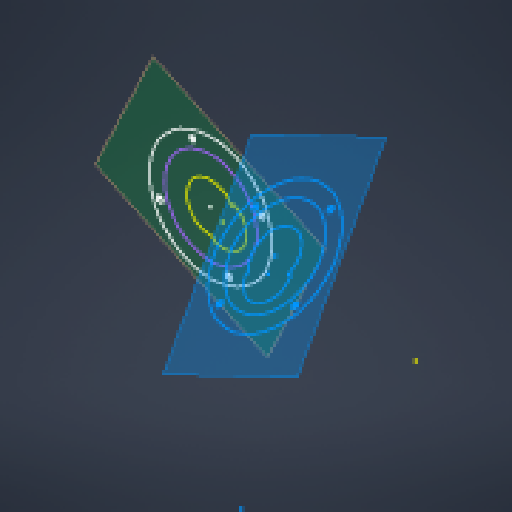
# Autodesk Inventor part: pylon_actuator_holder
Saved by Autodesk Inventor 2023.2 (Build 272271000, 271)
## iProperties
Created: 2023-07-02
Part Number: pylon_actuator_holder
Material: Generic
Document SubType Name: Modeling
Designer: Bober
Density: 1 g/cm^3
Appearance: Default
Author: Bober
Autodesk Inventor part; units mm, degrees
ref_plane "YZ Plane" through (0, 0, 0) normal (1, 0, 0) x (0, 1, 0)
ref_plane "XZ Plane" through (0, 0, 0) normal (0, 1, 0) x (-1, 0, 0)
ref_plane "XY Plane" through (0, 0, 0) normal (0, 0, 1) x (1, 0, 0)
ref_plane "Work Plane1" through (-137.7012, 21.7952, -38) normal (0, 0, -1) x (0.4270356, 0.9042348, 0)
sketch "Sketch1" plane through (-137.7012, 21.7952, -38) normal (0, 0, -1) x (0.4270356, 0.9042348, 0)
  arc A0 (-14.9525, 13.2962) -> (-14.999, 13.2194) centre (0, 4.2038) ccw projected
  arc A1 (14.999, 13.2194) -> (14.9525, 13.2962) centre (0, 4.2038) ccw projected
  circle A2 centre (0, 4.2038) radius 40 projected
  circle A3 centre (-24.7487, 28.9525) radius 2 projected
  circle A4 centre (24.7487, 28.9525) radius 2 projected
  circle A5 centre (24.7487, -20.5449) radius 2 projected
  circle A6 centre (-24.7487, -20.5449) radius 2 projected
  circle A7 centre (0, 4.2038) radius 40
  circle A8 centre (-24.7487, -20.5449) radius 2
  circle A9 centre (-24.7487, 28.9525) radius 2
  circle A10 centre (24.7487, 28.9525) radius 2
  circle A11 centre (24.7487, -20.5449) radius 2
  circle A12 centre (0, 4.2038) radius 30
  point P0 (39.0954, 133.8216)
  dimension "d0" = 3
  constraints: 6 centre point, 6 coincident, 5 concentric
ref_plane "Work Plane2" through (-187.1508, -33.2508, -28) normal (0, 0, 1) x (0.9042348, -0.4270356, 0)
extrude "Extrusion1" add sketch "Sketch1" against normal up to surface (10 mm away)
sketch "Sketch2" plane through (-133.9, 20, -28) normal (0, 0, 1) x (1, 0, 0)
  arc A0 (14.6069, 9.6378) -> (1.8364, -17.4034) centre (0, 0) ccw projected
  arc A1 (14.6069, 9.6378) -> (1.8364, -17.4034) centre (0, 0) ccw
  circle A2 centre (-8.3121, 3.9255) radius 6.025 projected
  arc A3 (10.5486, 1.0445) -> (5.8947, -8.81) centre (8.3121, -3.9255) ccw projected
  arc A4 (10.5486, 1.0445) -> (5.8947, -8.81) centre (8.3121, -3.9255) ccw
  line L0 (14.6069, 9.6378) -> (10.5486, 1.0445)
  line L1 (5.8947, -8.81) -> (1.8364, -17.4034)
  point P0 (133.9, -20)
  point P1 (5.8947, -8.81)
  point P2 (10.5486, 1.0445)
  point P3 (1.8364, -17.4034)
  point P4 (14.6069, 9.6378)
  point P5 (10.5486, 1.0445)
  point P6 (5.8947, -8.81)
  constraints: 4 end point, 4 point on circle, 2 centre point, 2 coincident, 2 concentric
ref_plane "Work Plane3" through (-157.1972, 0.2931, 0) normal (0, 0, 1) x (0.9042348, -0.4270356, 0)
ref_plane "Work Plane4" through (-157.1972, 0.2931, 0) normal (0, 0, 1) x (0.9042348, -0.4270356, 0)
extrude "Extrusion3" add sketch "Sketch2" along normal up to surface (28 mm away)
sketch "Sketch3" plane through (-133.9, 20, -28) normal (0, 0, 1) x (1, 0, 0)
  circle A0 centre (32.9473, 11.8101) radius 2 projected
  circle A1 centre (11.8101, -32.9473) radius 2 projected
  arc A2 (24.8559, 31.3398) -> (-8.4126, -39.1053) centre (0, 0) ccw
  line L0 (1.8364, -17.4034) -> (5.8947, -8.81) projected
  line L1 (1.8364, -17.4034) -> (-8.4126, -39.1053)
  line L2 (10.5486, 1.0445) -> (14.6069, 9.6378) projected
  line L3 (14.6069, 9.6378) -> (24.8559, 31.3398)
  circle A3 centre (0, 0) radius 40 projected
  circle A4 centre (-32.9473, -11.8101) radius 2 projected
  circle A5 centre (-11.8101, 32.9473) radius 2 projected
  arc A6 (10.5486, 1.0445) -> (5.8947, -8.81) centre (8.3121, -3.9255) ccw projected
  circle A7 centre (-8.3121, 3.9255) radius 6.025 projected
  point P0 (133.9, -20)
  constraints: 4 end point, 3 point on circle, 1 centre point, 1 coincident, 1 collinear, 1 point on line
extrude "Extrusion4" add sketch "Sketch3" along normal blind 5 contours L3 L2 A6 L0 L1 A2
thicken "Thicken1" operation add thickness 5 both sides no extend neighbours no toward (0, 0, 1) faces at (-137.8774, -16.2788, -28)
sketch "Sketch4" plane through (-133.9, 20, -23) normal (0, 0, 1) x (1, 0, 0)
  circle A0 centre (-11.8101, 32.9473) radius 2 projected
  circle A1 centre (-11.8101, 32.9473) radius 10
  circle A2 centre (-32.9473, -11.8101) radius 2 projected
  circle A3 centre (-32.9473, -11.8101) radius 10
  circle A4 centre (11.8101, -32.9473) radius 2 projected
  circle A5 centre (11.8101, -32.9473) radius 10
  circle A6 centre (32.9473, 11.8101) radius 2 projected
  circle A7 centre (32.9473, 11.8101) radius 10
  point P0 (133.9, -20)
  dimension "d11" = 20
  dimension "d12" = 20
  dimension "d13" = 20
  dimension "d14" = 20
  constraints: 4 centre point, 4 coincident
  measures "d11" diameter of A1
  measures "d12" diameter of A3
  measures "d13" diameter of A5
  measures "d14" diameter of A7
extrude "Extrusion5" cut sketch "Sketch4" against normal blind 3
sketch "Sketch5" plane through (-123.3514, 21.0445, 0) normal (0.9042348, -0.4270356, 0) x (0, 0, -1)
  circle A0 centre (24, 5.38) radius 1.5 projected
  circle A1 centre (24, -16.2782) radius 1.5 projected
  point P0 (0, 33.6463)
extrude "Extrusion6" cut sketch "Sketch5" against normal through all
ref_plane "Work Plane5" through (-141.4361, 29.5852, 0) normal (0.9042348, -0.4270356, 0) x (0, 0, -1)
sketch "Sketch6" plane through (-141.4361, 29.5852, 0) normal (0.9042348, -0.4270356, 0) x (0, 0, -1)
  circle A0 centre (24, 5.38) radius 1.5 projected
  line L0 (20.8246, 5.38) -> (22.4123, 8.13)
  line L1 (22.4123, 8.13) -> (25.5877, 8.13)
  line L2 (25.5877, 8.13) -> (27.1754, 5.38)
  line L3 (27.1754, 5.38) -> (25.5877, 2.63)
  line L4 (25.5877, 2.63) -> (22.4123, 2.63)
  line L5 (22.4123, 2.63) -> (20.8246, 5.38)
  circle A1 centre (24, -16.2782) radius 1.5 projected
  line L6 (22.4123, -19.0282) -> (20.8246, -16.2782)
  line L7 (20.8246, -16.2782) -> (22.4123, -13.5282)
  line L8 (22.4123, -13.5282) -> (25.5877, -13.5282)
  line L9 (25.5877, -13.5282) -> (27.1754, -16.2782)
  line L10 (27.1754, -16.2782) -> (25.5877, -19.0282)
  line L11 (25.5877, -19.0282) -> (22.4123, -19.0282)
  line L12 (23, 9.5035) -> (0, 9.5035) projected
  point P0 (0, 33.6463)
  dimension "d20" = 5.5
  dimension "d21" = 5.5
  constraints: 24 end point, 2 coincident, 2 parallel, 26 other
  measures "d20" distance between parallel lines of L1 L4
  measures "d21" distance between parallel lines of L8 L11
extrude "Extrusion7" cut sketch "Sketch6" against normal through all contours L0 L1 L2 L3 L4 L5 | A1 | L6 L7 L8 L9 L10 L11
body "Solid1"
